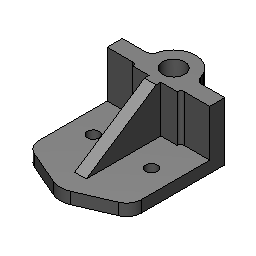
A3 v1 (Autodesk Fusion 360 design; units mm, degrees)
Autodesk Fusion 360 part; units mm, degrees
note: some values were not read from the file. Set by a fixed rule: which sketch regions a step uses.
sketch "Sketch1" plane through (0, 0, 0) normal (0, 0, 1) x (1, 0, 0)
  line L0 (44, 33.5) -> (-44, 33.5)
  line L1 (-44, 33.5) -> (-44, -33.5)
  line L2 (44, -33.5) -> (44, 33.5)
  circle A0 centre (-25, 2.5) radius 5
  circle A1 centre (25, 2.5) radius 5
  line L3 (-44, -33.5) -> (0, -52.5)
  line L4 (0, -52.5) -> (44, -33.5)
  dimension "d1" = 88
  dimension "d2" = 67
  dimension "d5" = 10
  dimension "d6" = 10
  dimension "d7" = 50
  dimension "d8" = 19
  dimension "d36" = 31
  constraint horizontal L0
  constraint perpendicular L0 L1
  constraint parallel L1 L2
  measures "d1" distance of L1.end L2.start
  measures "d2" distance of L0.end L1.end
  measures "d5" diameter of A0
  measures "d6" diameter of A1
  measures "d7" distance of A0.centre A1.centre
  measures "d8" distance of L2 A1.centre
  measures "d36" distance of L0 A1.centre
extrude "Extrude1" add sketch "Sketch1" along normal blind 10 makes body 1
fillet "Fillet2" radius 13 2 edges at (-44, -33.5, 5) (44, -33.5, 5) on bodies 1
fillet "Fillet3" radius 19 1 edges at (0, -52.5, 5) on bodies 1
sketch "Sketch2" plane through (0, 0, 10) normal (0, 0, 1) x (-1, 0, 0)
  arc A0 (7.5323, 49.2474) -> (-7.5323, 49.2474) centre (0, 31.8042) ccw
  line L0 (-7.5323, 49.2474) -> (-36.1537, 36.8882)
  arc A1 (-36.1537, 36.8882) -> (-44, 24.9534) centre (-31, 24.9534) ccw
  line L1 (-44, 24.9534) -> (-44, -33.5)
  line L2 (-44, -33.5) -> (44, -33.5)
  line L3 (44, -33.5) -> (44, 24.9534)
  arc A2 (44, 24.9534) -> (36.1537, 36.8882) centre (31, 24.9534) ccw
  line L4 (36.1537, 36.8882) -> (7.5323, 49.2474)
  circle A3 centre (25, -2.5) radius 5
  circle A4 centre (-25, -2.5) radius 5
  line L5 (-44, -33.5) -> (-44, -46.5)
  line L6 (44, -46.5) -> (44, -33.5)
  line L7 (-19, -33.5) -> (-19, -30.5)
  line L8 (19, -30.5) -> (19, -33.5)
  circle A5 centre (0, -46.5) radius 9.5
  line L9 (-5, -30.5) -> (-5, -26.5)
  line L10 (-5, -26.5) -> (5, -26.5)
  line L11 (5, -26.5) -> (5, -30.5)
  line L12 (-44, -46.5) -> (-19, -46.5)
  line L13 (19, -46.5) -> (44, -46.5)
  line L14 (44, -33.5) -> (19, -33.5)
  line L15 (-19, -33.5) -> (-44, -33.5)
  line L16 (-19, -30.5) -> (-5, -30.5)
  line L17 (5, -30.5) -> (19, -30.5)
  arc A6 (-19, -46.5) -> (19, -46.5) centre (0, -46.5) ccw
  dimension "d17" = 88
  dimension "d18" = 13
  dimension "d19" = 38
  dimension "d20" = 3
  dimension "d22" = 19
  dimension "d23" = 19
  dimension "d24" = 10
  dimension "d25" = 4
  constraint horizontal L14
  constraint vertical L5
  constraint horizontal L12
  constraint vertical L6
  constraint coincident L2.end L3.start
  constraint vertical L7
  constraint horizontal L16
  constraint vertical L8
  constraint coincident L2 L8.end
  constraint concentric A5 A6
  constraint vertical L9
  constraint horizontal L10
  constraint vertical L11
  constraint collinear L12 L13
  constraint coincident A5.centre L12
  constraint collinear L14 L15
  constraint collinear L16 L17
  measures "d17" distance of L2.end L1.end
  measures "d18" distance of L2.end L6.start
  measures "d19" distance of L8.end L7.start
  measures "d20" distance of L8.end L8.start
  measures "d22" radius of A6
  measures "d23" diameter of A5
  measures "d24" distance of L11.end L9.start
  measures "d25" distance of L11.end L10.end
extrude "Extrude2" add sketch "Sketch2" along normal blind 40 separate body contours L2 L5 L6 L12 L13 L14 L15 A6 | L2 L7 L8 L9 L10 L11 L16 L17 makes body 2
extrude "Extrude3" add 1 faces at (27.3333, 42.1667, 10) along direction (0, 0, -1) blind 10 on bodies 2 bodies 2 1
fillet "Fillet4" radius 3 2 edges at (-19, 33.5, 30) (19, 33.5, 30) on bodies 2
fillet "Fillet5" radius 6 2 edges at (19, 46.5, 25) (-19, 46.5, 25) on bodies 2
sketch "Sketch3" plane through (0, 0, 0) normal (1, 0, 0) x (0, 1, 0)
  line L0 (33.5239, 50) -> (33.5239, 10)
  line L1 (33.5239, 10) -> (-33.4761, 10)
  line L2 (26.5, 50) -> (-33.4761, 10)
  line L3 (26.5, 50) -> (33.5239, 50)
  dimension "d37" = 40
  dimension "d38" = 67
  constraint vertical L0
  constraint perpendicular L0 L1
  constraint perpendicular L0 L3
  measures "d37" distance of L0.start L0.end
  measures "d38" distance of L0.end L1.end
extrude "Extrude4" add sketch "Sketch3" along normal mid plane 10 bodies 2
named bodies: "A3"
